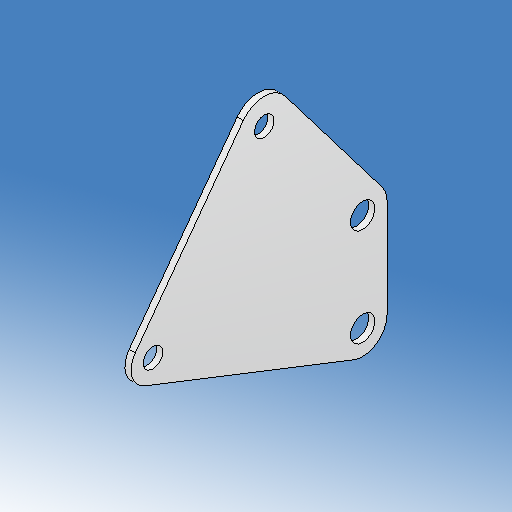
# Autodesk Inventor part: OuterDriveRail
Saved by Autodesk Inventor 2025 (Build 290162000, 162)
## iProperties
Created: 2023-02-06
Part Number: OuterDriveRail
Material: Aluminum 6061
Document SubType Name: Modeling
Designer: kumpu
Density: 2.7 g/cm^3
Appearance: Aluminum - Flat
Mass: 538.586 g
Surface Area: 696.12 cm^2
Volume: 199.476 cm^3
Author: kumpu
Autodesk Inventor part; units mm, degrees
(part 1 of 2)
ref_plane "YZ Plane" through (0, 0, 0) normal (1, 0, 0) x (0, 1, 0)
ref_plane "XZ Plane" through (0, 0, 0) normal (0, 1, 0) x (-1, 0, 0)
ref_plane "XY Plane" through (0, 0, 0) normal (0, 0, 1) x (1, 0, 0)
sketch "Sketch1" plane through (0, 0, 0) normal (1, 0, 0) x (0, 1, 0)
  line L0 (111.125, 190.5) -> (66.5265, 190.5)
  line L1 (19.3212, 158.834) -> (-11.1661, 102.5705)
  arc A0 (-11.1661, 102.5705) -> (-11.1661, 90.4695) centre (0, 96.52) ccw
  line L2 (-11.1661, 90.4695) -> (7.6076, 55.8231)
  arc A1 (-11.1661, 6.0505) -> (-11.1661, -6.0505) centre (0, 0) ccw
  line L3 (-11.1661, -6.0505) -> (7.6076, -40.6969)
  arc A2 (-11.1661, -90.4695) -> (-11.1661, -102.5705) centre (0, -96.52) ccw
  line L4 (-11.1661, -102.5705) -> (19.3212, -158.834)
  line L5 (66.5265, -190.5) -> (111.125, -190.5)
  line L6 (111.125, -190.5) -> (111.125, 190.5)
  arc A3 (19.3212, 158.834) -> (66.5265, 190.5) centre (41.275, 177.125) ccw
  arc A4 (66.5265, -190.5) -> (19.3212, -158.834) centre (41.275, -177.125) ccw
  circle A5 centre (73.5908, -125.0234) radius 6.35 construction
  line L7 (111.125, 0) -> (0, 0) construction
  circle A6 centre (0, 96.52) radius 2.4892 construction
  circle A7 centre (0, 0) radius 2.4892 construction
  circle A8 centre (0, -96.52) radius 2.4892 construction
  line L8 (-11.1661, 6.0505) -> (7.6076, 40.6969)
  arc A9 (7.6076, 40.6969) -> (7.6076, 55.8231) centre (-6.35, 48.26) ccw
  line L9 (-11.1661, -90.4695) -> (7.6076, -55.8231)
  arc A10 (7.6076, -55.8231) -> (7.6076, -40.6969) centre (-6.35, -48.26) ccw
  line L10 (-6.35, -48.26) -> (-6.35, 48.26) construction
  line L11 (-6.35, 0) -> (0, 0) construction
  circle A11 centre (0, 96.52) radius 3.175
  circle A12 centre (0, 0) radius 3.175
  circle A13 centre (0, -96.52) radius 3.175
  circle A14 centre (46.0375, 122.682) radius 3.5687 construction
  circle A15 centre (20.6375, 122.682) radius 3.5687 construction
  circle A16 centre (46.0375, 122.682) radius 3.175
  circle A17 centre (20.6375, 122.682) radius 3.175
  line L12 (0, 96.52) -> (-12.7, 96.52) construction
  circle A18 centre (99.3625, 57.3249) radius 2.0193
  circle A19 centre (48.3094, -33.0391) radius 2.0193
  circle A20 centre (99.3625, 31.9249) radius 2.0193
  circle A21 centre (73.9625, 57.3249) radius 2.0193
  circle A22 centre (73.9625, 31.9249) radius 2.0193
  circle A23 centre (48.3094, -58.4391) radius 2.0193
  circle A24 centre (22.9094, -33.0391) radius 2.0193
  circle A25 centre (22.9094, -58.4391) radius 2.0193
  circle A26 centre (85.725, 107.3629) radius 11
  line L13 (-12.7, 173.6352) -> (-12.7, -210.2893) construction
  circle A27 centre (85.725, 107.3629) radius 17.78 construction
  circle A28 centre (79.375, 147.5038) radius 22.86 construction
  circle A29 centre (41.275, 177.125) radius 25.4 construction
  line L14 (110.475, 71.2949) -> (60.975, 71.2949) construction
  line L15 (60.975, 71.2949) -> (60.975, -72.4091) construction
  line L16 (60.975, -72.4091) -> (110.475, -72.4091) construction
  line L17 (110.475, -72.4091) -> (110.475, 71.2949) construction
  line L18 (59.4219, 71.2949) -> (9.9219, 71.2949) construction
  line L19 (9.9219, 71.2949) -> (9.9219, -72.4091) construction
  line L20 (9.9219, -72.4091) -> (59.4219, -72.4091) construction
  line L21 (59.4219, -72.4091) -> (59.4219, 71.2949) construction
  line L22 (9.525, 127) -> (-15.875, 127) construction
  line L23 (-15.875, 127) -> (-15.875, -177.8) construction
  line L24 (-15.875, -177.8) -> (9.525, -177.8) construction
  line L25 (9.525, -177.8) -> (9.525, 127) construction
  circle A30 centre (34.6719, -108.4771) radius 17.78 construction
  circle A31 centre (41.275, -177.125) radius 31.75 construction
  circle A32 centre (102.0089, 180.2336) radius 2.413
  circle A33 centre (89.3089, 182.1987) radius 2.413
  circle A34 centre (102.0089, -180.2336) radius 2.413
  circle A35 centre (89.3089, -182.1987) radius 2.413
  circle A36 centre (79.375, 147.5038) radius 14.2875
  circle A37 centre (66.675, 254) radius 58.7375 construction
  circle A38 centre (66.675, -254) radius 58.7375 construction
  circle A39 centre (80.899, -155.6385) radius 47.527 construction
  circle A40 centre (92.075, -88.2841) radius 3.175
  circle A41 centre (66.675, -88.2841) radius 3.175
  circle A42 centre (92.075, -88.2841) radius 6.35 construction
  circle A43 centre (66.675, -88.2841) radius 6.35 construction
  circle A44 centre (46.0375, 122.682) radius 6.35 construction
  circle A45 centre (20.6375, 122.682) radius 6.35 construction
  circle A46 centre (17.4625, -132.7341) radius 3.175
  circle A47 centre (17.4625, -132.7341) radius 6.35 construction
  circle A48 centre (103.1875, 79.2324) radius 3.175
  circle A49 centre (103.1875, 79.2324) radius 6.35 construction
  line L26 (92.075, 107.3629) -> (79.375, 107.3629) construction
  line L27 (79.375, 107.3629) -> (79.375, 71.2949) construction
  line L28 (79.375, 71.2949) -> (92.075, 71.2949) construction
  line L29 (92.075, 71.2949) -> (92.075, 107.3629) construction
  line L30 (85.725, 107.3629) -> (85.725, 71.2949) construction
  circle A50 centre (71.4375, 79.2324) radius 3.175
  circle A51 centre (71.4375, 79.2324) radius 6.35 construction
  circle A52 centre (65.2528, -135.2431) radius 22.86 construction
  circle A53 centre (41.275, -177.125) radius 25.4 construction
  circle A54 centre (65.2528, -135.2431) radius 14.2875
  circle A55 centre (41.275, 177.125) radius 22.225 construction
  circle A56 centre (41.275, -177.125) radius 22.225 construction
  circle A57 centre (34.6719, -108.4771) radius 11
  circle A58 centre (79.375, 180.975) radius 3.175
  circle A59 centre (48.1711, 139.457) radius 3.175
  circle A60 centre (20.6375, 144.8678) radius 3.175
  circle A61 centre (79.375, 180.975) radius 6.35 construction
  circle A62 centre (48.1711, 139.457) radius 6.35 construction
  circle A63 centre (20.6375, 144.8678) radius 6.35 construction
  circle A64 centre (41.275, 177.125) radius 38.294 construction
  circle A65 centre (60.325, -104.1591) radius 3.175
  circle A66 centre (60.325, -104.1591) radius 6.35 construction
  point P0 (34.6719, -72.4091)
  dimension "d2" = 15.875
  dimension "d3" = 6.35
  dimension "d4" = 96.52
  dimension "d8" = 6.35
  dimension "d9" = 381
  dimension "d11" = 28.575
  dimension "d12" = 12.7
  dimension "d135" = 4.0386
  dimension "d136" = 4.0386
  dimension "d139" = 25.4
  dimension "d142" = 25.4
  dimension "d147" = 25.4
  dimension "d150" = 25.4
  dimension "d225" = 22
  dimension "d226" = 25.4
  dimension "d227" = 50.038
  dimension "d229" = 123.825
  dimension "d230" = 35.56
  dimension "d231" = 45.72
  dimension "d232" = 50.8
  dimension "d233" = 49.5
  dimension "d234" = 143.704
  dimension "d235" = 13.97
  dimension "d236" = 11.1125
  dimension "d237" = 143.704
  dimension "d238" = 49.5
  dimension "d239" = 11.1125
  dimension "d240" = 13.97
  dimension "d242" = 25.4
  dimension "d243" = 304.8
  dimension "d245" = 9.525
  dimension "d246" = 35.56
  dimension "d248" = 63.5
  dimension "d249" = 28.575
  dimension "d250" = 31.75
  dimension "d251" = 4.826
  dimension "d252" = 4.826
  dimension "d253" = 4.826
  dimension "d254" = 4.826
  dimension "d256" = 9.1161
  dimension "d257" = 12.7
  dimension "d258" = 1.9652
  dimension "d259" = 10.2664
  dimension "d260" = 12.7
  dimension "d261" = 1.9652
  dimension "d262" = 9.1161
  dimension "d263" = 10.2664
  dimension "d264" = 117.475
  dimension "d265" = 117.475
  dimension "d266" = 44.45
  dimension "d267" = 63.5
  dimension "d268" = 63.5
  dimension "d270" = 98.3615
  dimension "d271" = 14.224
  dimension "d272" = 95.054
  dimension "d273" = 6.35
  dimension "d274" = 6.35
  dimension "d275" = 25.4
  dimension "d276" = 19.05
  dimension "d277" = 12.7
  dimension "d278" = 12.7
  dimension "d279" = 12.7
  dimension "d280" = 12.7
  dimension "d283" = 6.35
  constraints: 62 end point, 61 centre point, 30 coincident, 18 point on circle, 17 tangent, 15 equal radius, 10 horizontal, 8 parallel, 6 midpoint, 5 perpendicular, 5 vertical, 2 horizontal alignment, 2 vertical alignment, 1 collinear, 1 equal length, 13 other
  measures "d2" radius of A9
  measures "d3" distance from line of L7.end L10
  measures "d4" distance of L10.start L10.end
  measures "d8" diameter of A11
  measures "d9" distance of L5.end L0.start
  measures "d11" radius of A3
  measures "d12" radius of A0
  measures "d135" diameter of A18
  measures "d136" diameter of A19
  measures "d139" distance of A18.centre A20.centre
  measures "d142" distance of A18.centre A21.centre
  measures "d147" distance of A19.centre A23.centre
  measures "d150" distance of A19.centre A24.centre
  measures "d225" diameter of A26
  measures "d226" distance from line of A26.centre L6
  measures "d227" vertical distance of A21.centre A26.centre
  measures "d229" distance between parallel lines of L13 L6
  measures "d230" diameter of A27
  measures "d231" diameter of A28
  measures "d232" diameter of A29
  measures "d233" distance of L15.end L16.end
  measures "d234" distance of L16.end L14.start
  measures "d235" distance from line of A18.centre L14
  measures "d236" distance from line of L17 A20.centre
  measures "d237" distance of L20.end L18.start
  measures "d238" distance of L18.start L18.end
  measures "d239" distance from line of L21 A23.centre
  measures "d240" distance from line of L20 A25.centre
  measures "d242" distance of L24.end L23.end
  measures "d243" distance of L22.end L23.end
  measures "d245" distance from line of A0.centre L25
  measures "d246" diameter of A30
  measures "d248" diameter of A31
  measures "d249" diameter of A36
  measures "d250" distance from line of A28.centre L6
  measures "d251" diameter of A32
  measures "d252" diameter of A33
  measures "d253" diameter of A34
  measures "d254" diameter of A35
  measures "d256" distance from line of A32.centre L6
  measures "d257" horizontal distance of A33.centre A32.centre
  measures "d258" vertical distance of A33.centre A32.centre
  measures "d259" distance from line of A32.centre L0
  measures "d260" horizontal distance of A35.centre A34.centre
  measures "d261" vertical distance of A35.centre A34.centre
  measures "d262" distance from line of L6 A34.centre
  measures "d263" distance from line of L5 A34.centre
  measures "d264" diameter of A37
  measures "d265" diameter of A38
  measures "d266" distance from line of A37.centre L6
  measures "d267" distance from line of L0 A37.centre
  measures "d268" distance from line of A38.centre L5
  measures "d270" vertical distance of A38.centre A39.centre
  measures "d271" horizontal distance of A38.centre A39.centre
  measures "d272" diameter of A39
  measures "d273" diameter of A41
  measures "d274" diameter of A40
  measures "d275" distance of A41.centre A40.centre
  measures "d276" distance from line of L6 A40.centre
  measures "d277" diameter of A43
  measures "d278" diameter of A42
  measures "d279" diameter of A44
  measures "d280" diameter of A45
  measures "d283" diameter of A46
extrude "Extrusion1" [suppressed]
sketch "Sketch2" plane through (12.7, 0, 0) normal (1, 0, 0) x (0, 0, -1)
  circle A0 centre (-96.52, 0) radius 3.175 construction
  line L0 (190.5, 111.125) -> (-190.5, 111.125) construction
  circle A1 centre (0, 0) radius 3.175 construction
  line L1 (0, 0) -> (0, 111.125) construction
  circle A2 centre (96.52, 0) radius 3.175 construction
  line L2 (96.52, 0) -> (96.52, 111.125) construction
  circle A3 centre (-122.682, 20.6375) radius 3.175 construction
  line L3 (-96.52, 0) -> (-122.682, 20.6375) construction
  circle A4 centre (-122.682, 46.0375) radius 3.175 construction
  line L4 (-122.682, 20.6375) -> (-122.682, 46.0375) construction
  circle A5 centre (-146.05, 85.725) radius 7.9375 construction
  line L5 (-122.682, 46.0375) -> (-146.05, 85.725) construction
  line L6 (-190.5, 111.125) -> (-190.5, 66.5265) construction
  line L7 (-146.05, 85.725) -> (-190.5, 111.125) construction
  line L8 (-146.05, 85.725) -> (-106.0351, 111.125) construction
  circle A6 centre (92.075, 34.925) radius 7.9375 construction
  circle A7 centre (125.0234, 73.5908) radius 6.35 construction
  line L9 (125.0234, 73.5908) -> (92.075, 34.925) construction
  line L10 (125.0234, 73.5908) -> (190.5, 111.125) construction
  line L11 (125.0234, 73.5908) -> (96.52, 111.125) construction
  circle A8 centre (69.85, 100.0125) radius 3.175 construction
  circle A9 centre (69.85, 74.6125) radius 3.175 construction
  line L12 (69.85, 100.0125) -> (69.85, 74.6125) construction
  line L13 (92.075, 34.925) -> (96.52, 0) construction
  line L14 (125.0234, 73.5908) -> (96.52, 0) construction
  line L15 (53.1812, 12.7) -> (53.1812, 57.15) construction
  line L16 (53.1812, 57.15) -> (53.1812, 111.125) construction
  line L17 (69.85, 100.0125) -> (53.1812, 111.125) construction
  line L18 (0, 0) -> (53.1812, 12.7) construction
  line L19 (0, 0) -> (-48.26, 10.3187) construction
  line L20 (-48.26, 10.3187) -> (-96.52, 0) construction
  line L21 (-48.26, 10.3187) -> (0, 111.125) construction
  line L22 (96.52, 0) -> (53.1812, 12.7) construction
  line L23 (-146.05, 85.725) -> (-122.682, 20.6375) construction
  line L24 (190.5, 66.5265) -> (190.5, 111.125) construction
  circle A10 centre (-190.5, 111.125) radius 3.9688 construction
  circle A11 centre (-96.52, 0) radius 3.9688 construction
  circle A12 centre (0, 0) radius 3.9688 construction
  circle A13 centre (96.52, 0) radius 3.9688 construction
  circle A14 centre (190.5, 111.125) radius 3.9688 construction
  circle A15 centre (0, 111.125) radius 3.9688 construction
  circle A16 centre (-146.05, 85.725) radius 3.9688 construction
  circle A17 centre (125.0234, 73.5908) radius 3.9688 construction
  circle A18 centre (92.075, 34.925) radius 3.9688 construction
  circle A19 centre (-48.26, 10.3187) radius 3.9688 construction
  circle A20 centre (-106.0351, 111.125) radius 3.9688 construction
  line L25 (-136.5891, 96.4312) -> (-119.693, 107.1562)
  line L26 (-119.693, 107.1562) -> (-167.6665, 107.1562)
  line L27 (-65.4177, 107.1562) -> (-6.3001, 107.1562)
  line L28 (-6.3001, 107.1562) -> (-48.5749, 18.852)
  line L29 (3.9688, 107.1562) -> (49.2625, 107.1562)
  line L30 (49.2625, 107.1562) -> (49.2625, 59.3278)
  line L31 (104.5173, 107.1562) -> (120.8881, 85.5986)
  line L32 (168.255, 107.1562) -> (104.5173, 107.1562)
  circle A21 centre (96.52, 111.125) radius 3.9688 construction
  circle A22 centre (69.85, 100.0125) radius 3.9688 construction
  circle A23 centre (69.85, 74.6125) radius 3.9688 construction
  line L33 (-132.3353, 89.7298) -> (-108.668, 104.7529)
  line L34 (-119.4185, 54.986) -> (-101.1904, 73.4311)
  circle A24 centre (-122.682, 46.0375) radius 3.9688 construction
  circle A25 centre (-122.682, 20.6375) radius 3.9688 construction
  circle A26 centre (-122.682, 46.0375) radius 9.525 construction
  line L35 (-3.9688, 93.644) -> (-42.0864, 14.0232)
  line L36 (-3.9688, 10.3796) -> (-3.9688, 93.644)
  line L37 (3.9688, 107.1562) -> (3.9688, 11.314)
  circle A27 centre (0, 0) radius 3.175 projected
  line L38 (73.7765, 65.9345) -> (112.3781, 74.7683)
  line L39 (77.1781, 80.6973) -> (96.4328, 104.6775)
  line L40 (96.4328, 104.6775) -> (114.5667, 80.7982)
  line L41 (63.9805, 55.55) -> (114.1488, 67.0308)
  line L42 (82.1272, 45.1805) -> (63.9805, 55.55)
  line L43 (89.8709, 20.8085) -> (91.2725, 9.7955)
  line L44 (-122.682, 46.0375) -> (-76.4287, 92.8415) construction
  line L45 (-190.5, 111.125) -> (-190.5, -12.7)
  line L46 (-190.5, -12.7) -> (190.5, -12.7)
  line L47 (190.5, -12.7) -> (190.5, 111.125)
  arc A28 (-6.0505, -11.1661) -> (6.0505, -11.1661) centre (0, 0) ccw construction
  arc A29 (-136.5891, 96.4312) -> (-156.4804, 95.4891) centre (-146.05, 85.725) ccw
  arc A30 (-131.772, 86.2463) -> (-132.3353, 89.7298) centre (-146.05, 85.725) ccw
  arc A31 (-190.5, 111.125) -> (-184.6538, 104.795) centre (-184.15, 111.125) ccw
  arc A32 (-160.0618, 82.9318) -> (-184.6538, 104.795) centre (-186.8185, 77.5979) ccw
  arc A33 (-160.0618, 82.9318) -> (-153.0864, 73.2903) centre (-146.05, 85.725) ccw
  arc A34 (-131.8934, 23.0615) -> (-153.0864, 73.2903) centre (-175.0785, 34.4258) ccw
  arc A35 (-119.4185, 54.986) -> (-126.5651, 54.735) centre (-122.682, 46.0375) ccw
  arc A36 (-131.8934, 23.0615) -> (-118.8104, 11.9348) centre (-122.682, 20.6375) ccw
  arc A37 (-156.4804, 95.4891) -> (-167.6665, 107.1562) centre (-186.8185, 77.5979) ccw
  arc A38 (-126.5651, 54.735) -> (-139.486, 73.1451) centre (-175.0785, 34.4258) ccw
  arc A39 (-139.486, 73.1451) -> (-133.8392, 78.5818) centre (-146.192, 85.761) ccw
  line L48 (-96.52, 0) -> (0, 0) construction
  line L49 (-48.26, 0) -> (-48.26, 6.35) construction
  arc A40 (-107.3496, 2.4916) -> (-118.8104, 11.9348) centre (-115.4372, 4.3524) ccw
  arc A41 (-107.3496, 2.4916) -> (-89.4091, -8.5395) centre (-96.52, 0) ccw
  arc A42 (-7.1109, -8.5395) -> (-89.4091, -8.5395) centre (-48.26, -57.9553) ccw
  arc A43 (-7.1109, -8.5395) -> (7.1109, -8.5395) centre (0, 0) ccw
  arc A44 (89.4091, -8.5395) -> (7.1109, -8.5395) centre (48.26, -57.9553) ccw
  arc A45 (89.4091, -8.5395) -> (107.4129, 2.1985) centre (96.52, 0) ccw
  arc A46 (132.1844, 63.1022) -> (107.4129, 2.1985) centre (165.7303, 13.9684) ccw
  arc A47 (185.7041, 104.9681) -> (190.5, 111.125) centre (184.15, 111.125) ccw
  arc A48 (185.7041, 104.9681) -> (136.0465, 67.2834) centre (205.2058, 27.7108) ccw
  arc A49 (132.1844, 63.1022) -> (136.0465, 67.2834) centre (125.0234, 73.5908) ccw
  arc A50 (-86.0187, 3.6345) -> (-88.1432, 7.3019) centre (-96.52, 0) ccw
  arc A51 (-3.9688, 10.3796) -> (-10.5013, 3.6345) centre (0, 0) ccw
  arc A52 (-10.5013, 3.6345) -> (-42.0864, 14.0232) centre (-48.26, -57.9553) ccw
  arc A53 (-53.8119, 14.0739) -> (-86.0187, 3.6345) centre (-48.26, -57.9553) ccw
  arc A54 (10.5013, 3.6345) -> (9.5832, 5.6259) centre (0, 0) ccw
  arc A55 (39.4872, 13.7529) -> (10.5013, 3.6345) centre (48.26, -57.9553) ccw
  arc A56 (86.0187, 3.6345) -> (47.4247, 14.2827) centre (48.26, -57.9553) ccw
  arc A57 (91.2725, 9.7955) -> (86.0187, 3.6345) centre (96.52, 0) ccw
  arc A58 (135.4904, 80.7834) -> (120.8881, 85.5986) centre (125.0234, 73.5908) ccw
  arc A59 (168.255, 107.1562) -> (135.4904, 80.7834) centre (205.2058, 27.7108) ccw
  arc A60 (73.7765, 65.9345) -> (77.1781, 80.6973) centre (69.85, 74.6125) ccw
  arc A61 (114.5667, 80.7982) -> (112.3781, 74.7683) centre (125.0234, 73.5908) ccw
  arc A62 (101.052, 46.0401) -> (82.1272, 45.1805) centre (92.075, 34.925) ccw
  arc A63 (79.7883, 42.2168) -> (80.2054, 26.9722) centre (92.075, 34.925) ccw
  arc A64 (80.2054, 26.9722) -> (89.8709, 20.8085) centre (92.075, 34.925) ccw
  arc A65 (114.1488, 67.0308) -> (115.2054, 65.5349) centre (125.0234, 73.5908) ccw
  arc A66 (115.2054, 65.5349) -> (101.052, 46.0401) centre (165.7303, 13.9684) ccw
  circle A67 centre (-57.3249, 99.3625) radius 2.0193 construction
  circle A68 centre (-57.3249, 73.9625) radius 2.0193 construction
  circle A69 centre (-31.9249, 99.3625) radius 2.0193 construction
  circle A70 centre (-31.9249, 73.9625) radius 2.0193 construction
  circle A71 centre (58.4391, 22.9094) radius 2.0193 construction
  circle A72 centre (33.0391, 22.9094) radius 2.0193 construction
  circle A73 centre (33.0391, 48.3094) radius 2.0193 construction
  circle A74 centre (58.4391, 48.3094) radius 2.0193 construction
  line L50 (-106.0351, 111.125) -> (-81.6196, 80.1887) construction
  line L51 (-96.012, 99.3625) -> (-96.012, 73.9625) construction
  line L52 (-57.3249, 73.025) -> (-31.9249, 73.025) construction
  line L53 (-70.612, 73.9625) -> (-70.612, 99.3625) construction
  line L54 (-31.9249, 98.425) -> (-57.3249, 98.425) construction
  line L55 (-146.192, 85.761) -> (-59.8898, 63.8569) construction
  line L56 (-96.0036, 74.2316) -> (-96.52, 0) construction
  line L57 (-96.52, 0) -> (-65.9914, 86.0487) construction
  circle A75 centre (-57.3249, 99.3625) radius 5.1943
  circle A76 centre (-70.612, 98.425) radius 5.1943
  circle A77 centre (-96.012, 73.025) radius 5.1943
  circle A78 centre (-70.612, 73.025) radius 5.1943
  circle A79 centre (33.0391, 48.3094) radius 5.1943
  circle A80 centre (43.18, 47.625) radius 5.1943
  circle A81 centre (17.78, 22.225) radius 5.1943
  circle A82 centre (43.18, 22.225) radius 5.1943
  line L58 (-70.612, 73.025) -> (-48.26, 10.3187) construction
  line L59 (-99.4531, 94.4823) -> (-108.668, 104.7529)
  line L60 (-133.8392, 78.5818) -> (-100.2798, 70.0642)
  line L61 (-131.772, 86.2463) -> (-98.2146, 77.7292)
  line L62 (-77.1372, 79.5502) -> (-70.612, 73.025) construction
  line L63 (-92.6609, 76.9937) -> (-73.9631, 76.9937)
  line L64 (-92.6609, 69.0562) -> (-73.9631, 69.0562)
  line L65 (-74.5808, 95.0739) -> (-74.5808, 76.3761)
  line L66 (-66.6433, 95.0739) -> (-66.6433, 76.3761)
  line L67 (-99.9808, 95.0739) -> (-99.9808, 76.3761)
  line L68 (-92.0433, 95.0739) -> (-92.0433, 76.3761)
  line L69 (-92.6609, 94.4562) -> (-73.9631, 94.4562)
  line L70 (-92.6609, 102.3937) -> (-73.9631, 102.3937)
  line L71 (-96.4488, 93.2491) -> (-75.7879, 72.5882)
  line L72 (-90.8361, 98.8618) -> (-70.1752, 78.2009)
  line L73 (-113.7728, 49.4066) -> (-95.5446, 67.8518)
  line L74 (-73.2252, 68.5359) -> (-53.8119, 14.0739)
  line L75 (-65.7485, 71.201) -> (-47.7228, 20.6319)
  line L76 (-89.3091, 8.4552) -> (-67.9922, 68.5398)
  line L77 (-96.7898, 11.1092) -> (-75.4728, 71.1938)
  line L78 (-100.2104, 20.4213) -> (-100.2104, 69.9665)
  line L79 (-92.4791, 10.3518) -> (-92.0667, 69.6464)
  line L80 (-113.5349, 43.3812) -> (-100.2104, 20.4213)
  arc A83 (-113.5349, 43.3812) -> (-113.7728, 49.4066) centre (-122.682, 46.0375) ccw
  circle A84 centre (-96.52, 0) radius 11.1125 construction
  arc A85 (-88.1432, 7.3019) -> (-89.3091, 8.4552) centre (-96.52, 0) ccw
  line L81 (-65.4177, 107.1562) -> (-65.4177, 98.425)
  line L82 (17.78, 22.225) -> (43.18, 22.225) construction
  line L83 (43.18, 22.225) -> (43.18, 47.625) construction
  line L84 (43.18, 47.625) -> (33.0391, 47.625) construction
  line L85 (17.78, 48.3094) -> (17.78, 22.225) construction
  line L86 (25.0718, 40.3375) -> (43.1946, 22.225) construction
  line L87 (17.78, 22.225) -> (0, 0) construction
  line L88 (69.85, 74.6125) -> (43.18, 47.625) construction
  line L89 (92.075, 34.925) -> (43.18, 47.625) construction
  line L90 (92.075, 34.925) -> (43.1946, 22.225) construction
  line L91 (21.1311, 51.5938) -> (39.8289, 51.5938)
  line L92 (21.1311, 43.6563) -> (39.8289, 43.6563)
  line L93 (13.8112, 44.2739) -> (13.8112, 25.4502)
  line L94 (12.5875, 22.0875) -> (-3.0991, 2.4793)
  line L95 (18.7857, 17.129) -> (3.0991, -2.4793)
  line L96 (21.1311, 18.2563) -> (39.8289, 18.2563)
  line L97 (21.1311, 26.1938) -> (39.8289, 26.1938)
  line L98 (39.2112, 25.5761) -> (39.2112, 44.2739)
  line L99 (47.1487, 25.5761) -> (47.1487, 44.2739)
  line L100 (43.6313, 27.3997) -> (22.9558, 48.0632)
  line L101 (38.0029, 21.8027) -> (17.3447, 42.449)
  line L102 (67.0195, 77.3945) -> (42.8556, 52.8092)
  line L103 (48.3446, 47.0702) -> (72.6805, 71.8305)
  line L104 (45.4257, 42.9413) -> (77.7928, 34.5342)
  line L105 (47.4212, 50.6238) -> (79.7883, 42.2168) construction
  line L106 (46.5311, 18.2563) -> (80.1865, 27.0005)
  line L107 (45.4305, 26.9064) -> (77.7928, 35.3147)
  line L108 (21.7487, 44.2739) -> (21.7487, 25.5761)
  line L109 (14.4289, 51.5938) -> (3.9688, 51.5938)
  line L110 (14.4289, 43.6563) -> (3.9688, 43.6563)
  line L111 (33.0391, 47.625) -> (0, 47.625) construction
  line L112 (39.4872, 18.5721) -> (39.4872, 8.9337)
  line L113 (47.4247, 19.2311) -> (47.4247, 9.3342)
  point P0 (-104.0605, 99.6176)
  point P1 (-83.312, 76.9937)
  point P2 (-74.5808, 85.725)
  point P3 (-104.6587, 58.6292)
  point P4 (-110.3045, 64.2086)
  point P5 (-109.347, 59.5312)
  point P6 (-92.2729, 39.9991)
  point P7 (-103.6679, 70.9241)
  point P8 (-70.6032, 61.1802)
  point P9 (-92.0708, 69.0562)
  point P10 (-92.3876, 23.5174)
  point P11 (-76.2312, 69.0562)
  point P12 (-100.2104, 63.1305)
  point P13 (-99.9808, 78.1775)
  point P14 (-99.9808, 95.0704)
  point P15 (-86.4306, 94.4562)
  point P16 (-74.5808, 82.6064)
  point P17 (-74.5808, 94.4562)
  point P18 (-80.1934, 76.9937)
  point P19 (-92.0433, 88.8436)
  point P20 (-92.0433, 76.9937)
  point P21 (30.48, 51.5938)
  point P22 (33.2935, 37.7315)
  point P23 (39.2112, 34.925)
  point P24 (9.1988, 43.6563)
  point P25 (0, 47.625)
  point P26 (47.1487, 27.3529)
  point P27 (76.2905, 34.9244)
  point P28 (47.1487, 42.4937)
  point P29 (39.4872, 18.2563)
  point P30 (27.3653, 43.6563)
  point P31 (39.2112, 31.8171)
  point P32 (39.2112, 43.6563)
  point P33 (21.7487, 38.0475)
  point P34 (21.7487, 26.1938)
  point P35 (33.6093, 26.1938)
  point P36 (13.8112, 43.6563)
  point P37 (13.8112, 25.5761)
  point P38 (47.4247, 18.4884)
  dimension "d17" = 19.05
  dimension "d65" = 12.7
  dimension "d13" = 44.45
  dimension "d14" = 7.9375
  dimension "d29" = 14.2875
  dimension "d30" = 9.525
  dimension "d31" = 6.35
  dimension "d32" = 7.9375
  dimension "d33" = 7.9375
  dimension "d34" = 6.35
  dimension "d35" = 11.1125
  dimension "d36" = 12.7
  dimension "d37" = 7.9375
  dimension "d38" = 7.9375
  dimension "d39" = 7.9375
  dimension "d40" = 12.7
  dimension "d157" = 3.175
  dimension "d160" = 25.4
  dimension "d163" = 25.4
  dimension "d166" = 3.175
  dimension "d169" = 25.4
  dimension "d172" = 25.4
  dimension "d177" = 7.9375
  dimension "d180" = 7.9375
  dimension "d181" = 3.9688
  dimension "d182" = 7.9375
  dimension "d183" = 3.9688
  dimension "d185" = 7.9375
  dimension "d186" = 3.9688
  dimension "d187" = 7.9375
  dimension "d188" = 3.9688
  dimension "d189" = 7.9375
  dimension "d190" = 3.9688
  dimension "d191" = 7.9375
  dimension "d192" = 3.9688
  dimension "d194" = 7.9375
  dimension "d195" = 7.9375
  dimension "d196" = 3.9688
  dimension "d197" = 3.9688
  dimension "d198" = 7.9375
  dimension "d199" = 3.9688
  dimension "d202" = 7.9375
  dimension "d203" = 0.156
  dimension "d204" = 7.9375
  dimension "d205" = 3.9688
  dimension "d206" = 7.9375
  dimension "d207" = 3.9688
  dimension "d208" = 7.9375
  dimension "d209" = 3.9688
  dimension "d210" = 7.9375
  dimension "d211" = 7.9375
  dimension "d212" = 3.9688
  dimension "d213" = 3.9688
  dimension "d214" = 3.9688
  dimension "d215" = 8.649
  dimension "d216" = 3.9688
  dimension "d217" = 7.9375
  dimension "d218" = 3.9688
  dimension "d220" = 7.9375
  dimension "d221" = 7.9375
  dimension "d222" = 3.9688
  dimension "d223" = 7.9375
  constraints: 222 end point, 104 point on circle, 59 centre point, 42 tangent, 33 concentric, 33 parallel, 28 coincident, 22 equal radius, 18 vertical, 14 midpoint, 14 point on line, 13 horizontal, 13 perpendicular, 3 collinear, 2 line through centre, 1 equal length, 82 other
  measures "d13" distance of L15.start L15.end
  measures "d14" diameter of A10
  measures "d29" radius of A29
  measures "d30" radius of A35
  measures "d31" radius of A31
  measures "d32" radial gap between concentric circles of A32 A37
  measures "d33" radial gap between concentric circles of A34 A38
  measures "d34" distance of L49.start L49.end
  measures "d35" radius of A41
  measures "d36" radius of A49
  measures "d37" radial gap between concentric circles of A42 A53
  measures "d38" radial gap between concentric circles of A44 A55
  measures "d39" radial gap between concentric circles of A48 A59
  measures "d40" radial gap between concentric circles of A46 A66
  measures "d177" distance between parallel lines of L61 L60
  measures "d180" distance from line of L64 point (-83.312, 76.994)
  measures "d181" distance between parallel lines of L63 L52
  measures "d182" distance between parallel lines of L66 L65
  measures "d183" distance from line of point (-74.581, 85.725) L53
  measures "d185" distance between parallel lines of L68 L67
  measures "d186" distance between parallel lines of L67 L51
  measures "d187" distance between parallel lines of L69 L70
  measures "d188" distance between parallel lines of L54 L70
  measures "d189" distance between parallel lines of L72 L71
  measures "d190" distance between parallel lines of L62 L71
  measures "d191" distance of point (-104.659, 58.629) point (-110.304, 64.209)
  measures "d192" distance from line of L73 point (-109.347, 59.531)
  measures "d194" distance from line of point (-92.273, 39.999) L78
  measures "d195" distance between parallel lines of L76 L77
  measures "d196" distance between parallel lines of L79 L56
  measures "d197" distance between parallel lines of L76 L57
  measures "d198" distance between parallel lines of L75 L74
  measures "d199" distance between parallel lines of L58 L74
  measures "d202" distance between parallel lines of L103 L102
  measures "d203" angle of L102 L88
  measures "d204" distance from line of L92 point (30.48, 51.594)
  measures "d205" distance between parallel lines of L91 L84
  measures "d206" distance between parallel lines of L100 L101
  measures "d207" distance from line of point (33.294, 37.731) L86
  measures "d208" distance between parallel lines of L108 L93
  measures "d209" distance between parallel lines of L108 L85
  measures "d210" distance from line of L99 point (39.211, 34.925)
  measures "d211" distance between parallel lines of L96 L97
  measures "d212" distance between parallel lines of L82 L96
  measures "d213" distance between parallel lines of L99 L83
  measures "d214" distance between parallel lines of L107 L90
  measures "d215" distance between parallel lines of L107 L106
  measures "d216" distance between parallel lines of L89 L104
  measures "d217" distance between parallel lines of L105 L104
  measures "d218" distance between parallel lines of L87 L94
  measures "d220" distance between parallel lines of L95 L94
  measures "d221" distance from line of L109 point (9.199, 43.656)
  measures "d222" distance between parallel lines of L110 L111
  measures "d223" horizontal distance of A56.end A55.start
extrude "Extrusion2" [suppressed]
delete_face "Delete Face1" [suppressed]
fillet "Fillet1" [suppressed]
fillet "Fillet2" [suppressed]
fillet "Fillet3" [suppressed]
sketch "Sketch4" plane through (0, 111.125, 190.5) normal (0, 1, 0) x (1, 0, 0)
  line L0 (12.7, 281.8419) -> (12.7, 291.8504) projected
  line L1 (12.7, 346.4492) -> (12.7, 349.6242) projected
  line L2 (12.7, 26.0204) -> (12.7, 27.6079) projected
  line L3 (12.7, 381) -> (12.7, 0) projected
  line L4 (12.7, 18.9559) -> (0, 18.9559)
  line L5 (12.7, 87.1601) -> (0, 87.1601)
  line L6 (0, 381) -> (0, 0) projected
  line L7 (12.7, 190.5) -> (0, 190.5)
  line L8 (12.7, 274.2219) -> (0, 274.2219)
  line L9 (12.7, 357.5617) -> (0, 357.5617)
  circle A0 centre (6.35, 18.9559) radius 3.175
  circle A1 centre (6.35, 87.1601) radius 3.175
  circle A2 centre (6.35, 190.5) radius 3.175
  circle A3 centre (6.35, 274.2219) radius 3.175
  circle A4 centre (6.35, 357.5617) radius 3.175
  point P0 (12.7, 194.4688)
  point P1 (12.7, 186.5313)
  point P2 (12.7, 80.518)
  point P3 (12.7, 94.0577)
  point P4 (12.7, 348.1717)
  point P5 (12.7, 26.5759)
  point P6 (12.7, 348.0367)
  dimension "d42" = 9.525
  dimension "d43" = 7.62
  dimension "d44" = 6.6421
  dimension "d45" = 7.62
  dimension "d46" = 6.35
  dimension "d47" = 6.35
  dimension "d48" = 6.35
  dimension "d49" = 6.35
  dimension "d50" = 6.35
  constraints: 10 end point, 6 midpoint, 5 centre point, 3 horizontal, 2 point on line, 1 parallel, 1 perpendicular, 6 other
  measures "d42" distance from line of point (12.7, 348.037) L9
  measures "d43" distance from line of L0.start L8
  measures "d44" distance from line of L5 point (12.7, 80.518)
  measures "d45" distance from line of point (12.7, 26.576) L4
  measures "d46" diameter of A0
  measures "d47" diameter of A1
  measures "d48" diameter of A2
  measures "d49" diameter of A3
  measures "d50" diameter of A4
extrude "Extrusion4" [suppressed]
thread "Thread1" size "1/4-20 UNC" class "2B" standard "ANSI Unified Screw Threads" full length
thread "Thread2" size "1/4-20 UNC" class "2B" standard "ANSI Unified Screw Threads" full length
thread "Thread3" size "1/4-20 UNC" class "2B" standard "ANSI Unified Screw Threads" full length
thread "Thread4" size "1/4-20 UNC" class "2B" standard "ANSI Unified Screw Threads" full length
thread "Thread5" size "1/4-20 UNC" class "2B" standard "ANSI Unified Screw Threads" full length
sketch "Sketch5" plane through (12.7, 111.125, 190.5) normal (1, 0, 0) x (0, 0, -1)
  arc A0 (0, 0) -> (5.8462, -6.33) centre (6.35, 0) ccw projected
  arc A1 (30.4382, -28.1932) -> (37.4136, -37.8347) centre (44.45, -25.4) ccw projected
  arc A2 (58.6066, -88.0635) -> (37.4136, -37.8347) centre (15.4215, -76.6992) ccw projected
  spline S0 degree 4 poles (0, 0) (0, -17.1941) (-2.2287, -33.2158) (22.5292, -29.4121) (37.4136, -37.8347) knots 0 0 0 0 0 1 1 1 1 1
  line L0 (0, 8.2432) -> (0, -8.2432) construction
  arc A3 (-0.1228, -6.59) -> (-0.1228, 6.59) centre (-176.868, 0) ccw construction
  line L1 (31.1102, -34.2678) -> (43.7171, -41.4016) construction
  arc A4 (42.0116, -41.1741) -> (32.1834, -35.6126) centre (25.0253, -59.7274) ccw construction
  arc A5 (30.4382, -28.1932) -> (5.8462, -6.33) centre (3.6815, -33.5271) ccw projected
  point P0 (190.5, -111.125)
  point P1 (5.8462, -25.4)
  constraints: 4 end point, 4 midpoint, 2 centre point, 2 point on circle, 2 vertical, 1 tangent, 6 other
extrude "Extrusion5" [suppressed]
sketch "Sketch6" plane through (12.7, -57.9553, 48.26) normal (1, 0, 0) x (0, 0, -1)
  arc A0 (-123.1359, 156.0289) -> (-125.9731, 144.465) centre (-97.79, 143.6803) ccw
  line L0 (-122.8964, 163.3325) -> (-122.523, 159.4124)
  line L1 (-142.24, 169.0803) -> (-129.2178, 169.0803)
  spline S0 degree 2 poles (-221.2962, 144.7093) (-189.8396, 169.0803) (-142.24, 169.0803) knots 1 1 1 2 2 2
  arc A1 (-221.2962, 144.7093) -> (-187.7795, 106.6698) centre (-205.74, 124.6303) ccw
  circle A2 centre (-133.9387, 147.2642) radius 6.35
  line L2 (-141.6133, 153.8382) -> (-140.1827, 146.1086)
  line L3 (-135.7752, 141.1856) -> (-124.621, 137.8157)
  line L4 (238.76, 169.0803) -> (-142.24, 169.0803)
  circle A3 centre (144.78, 57.9553) radius 3.175
  circle A4 centre (-48.26, 57.9553) radius 3.175
  circle A5 centre (48.26, 57.9553) radius 3.175
  circle A6 centre (-74.422, 103.9928) radius 3.175
  circle A7 centre (-74.422, 78.5928) radius 3.175
  spline S1 degree 3 poles (-159.7966, 136.4204) (-160.5161, 136.0307) (-162.9434, 134.6743) (-166.1744, 132.6857) (-170.3078, 129.9138) (-173.1321, 127.8669) (-175.1101, 126.3517) (-175.4939, 126.0547) knots 0 0 0 0 0.132459 0.448869 0.607074 0.923484 1 1 1 1
  spline S2 degree 3 poles (-180.582, 128.1282) (-180.5251, 127.7187) (-180.3887, 127.3243) (-179.9724, 126.6098) (-179.6965, 126.2967) (-179.0402, 125.7938) (-178.666, 125.6088) (-177.8679, 125.3927) (-177.4515, 125.3637) (-176.7607, 125.4505) (-176.4861, 125.5231) (-175.9633, 125.7391) (-175.7175, 125.8816) (-175.4939, 126.0547) knots 0 0 0 0 0.12403 0.12403 0.248059 0.248059 0.372089 0.372089 0.496118 0.496118 0.580963 0.580963 0.665808 0.665808 0.665808 0.665808
  arc A8 (-180.582, 128.1282) -> (-185.3963, 139.8386) centre (-205.74, 124.6303) ccw
  arc A9 (-182.4834, 144.893) -> (-185.3963, 139.8386) centre (-182.8533, 141.7397) ccw
  line L5 (-182.4834, 144.893) -> (-160.9387, 142.3656)
  spline S3 degree 3 poles (-159.7966, 136.4204) (-159.4331, 136.6173) (-159.1114, 136.8833) (-158.5883, 137.5236) (-158.3918, 137.8918) (-158.1509, 138.6828) (-158.1089, 139.0981) (-158.1864, 139.9213) (-158.3051, 140.3214) (-158.6893, 141.0536) (-158.9511, 141.3786) (-159.5039, 141.8425) (-159.7675, 142.0051) (-160.3334, 142.2494) (-160.6326, 142.3297) (-160.9387, 142.3656) knots 0 0 0 0 0.12403 0.12403 0.248059 0.248059 0.372089 0.372089 0.496118 0.496118 0.620148 0.620148 0.712599 0.712599 0.80505 0.80505 0.80505 0.80505
  line L6 (-150.5941, 147.5473) -> (-181.7868, 151.2066)
  spline S4 degree 3 poles (-182.3079, 157.4074) (-182.7047, 157.2914) (-183.0751, 157.099) (-183.7212, 156.583) (-183.9908, 156.2643) (-184.3926, 155.5417) (-184.521, 155.1446) (-184.6185, 154.3235) (-184.5865, 153.9073) (-184.3649, 153.1107) (-184.1773, 152.7379) (-183.6699, 152.085) (-183.3548, 151.8113) (-182.8106, 151.4993) (-182.6148, 151.4119) (-182.2086, 151.2779) (-181.9992, 151.2315) (-181.7868, 151.2066) knots 0 0 0 0 0.12403 0.12403 0.248059 0.248059 0.372089 0.372089 0.496118 0.496118 0.620148 0.620148 0.744178 0.744178 0.808342 0.808342 0.872507 0.872507 0.872507 0.872507
  spline S5 degree 3 poles (-182.3079, 157.4074) (-181.8014, 157.5555) (-180.2373, 158.0014) (-176.5127, 158.9811) (-172.1175, 159.9481) (-165.3484, 161.1597) (-158.303, 162.0566) (-152.1732, 162.4641) (-149.655, 162.5727) knots 0 0 0 0 0.050647 0.155729 0.365894 0.470976 0.786223 1 1 1 1
  spline S6 degree 3 poles (-146.3536, 159.1439) (-146.3201, 159.5559) (-146.3675, 159.9706) (-146.6185, 160.7584) (-146.8198, 161.1241) (-147.3511, 161.7576) (-147.6761, 162.0195) (-148.2892, 162.3414) (-148.5523, 162.438) (-149.097, 162.5599) (-149.3762, 162.5847) (-149.655, 162.5727) knots 0 0 0 0 0.12403 0.12403 0.248059 0.248059 0.372089 0.372089 0.45581 0.45581 0.539531 0.539531 0.539531 0.539531
  line L7 (-146.3536, 159.1439) -> (-147.0595, 150.4439)
  arc A10 (-150.5941, 147.5473) -> (-147.0595, 150.4439) centre (-150.2241, 150.7007) ccw
  arc A11 (-122.8964, 163.3325) -> (-129.2178, 169.0803) centre (-129.2178, 162.7303) ccw
  spline S7 degree 3 poles (-125.9731, 144.465) (-125.9961, 143.6384) (-126.1803, 142.8243) (-126.8505, 141.3124) (-127.33, 140.6292) (-128.4917, 139.516) (-129.1514, 139.0838) (-130.5947, 138.4809) (-131.3658, 138.3154) (-132.1476, 138.2941) knots 0 0 0 0 0.248059 0.248059 0.496118 0.496118 0.730735 0.730735 0.965351 0.965351 0.965351 0.965351
  arc A12 (-123.1359, 156.0289) -> (-122.523, 159.4124) centre (-128.8444, 158.8102) ccw
  spline S8 degree 3 poles (-132.1476, 138.2941) (-151.3774, 137.7699) (-171.7443, 122.7049) (-187.7795, 106.6698) knots 0.172109 0.172109 0.172109 0.172109 1 1 1 1
  circle A13 centre (-205.74, 124.6303) radius 15.24
  circle A14 centre (-133.9387, 147.2642) radius 1.27
  circle A15 centre (-131.9736, 159.9642) radius 1.27
  circle A16 centre (81.2991, 80.8647) radius 2.0193
  line L8 (-142.24, 169.0803) -> (-142.24, 124.4818)
  arc A17 (-110.574, 77.2765) -> (-142.24, 124.4818) centre (-128.865, 99.2303) ccw
  line L9 (-110.574, 77.2765) -> (-54.3105, 46.7892)
  arc A18 (-54.3105, 46.7892) -> (-42.2095, 46.7892) centre (-48.26, 57.9553) ccw
  line L10 (-42.2095, 46.7892) -> (-7.5631, 65.5629)
  arc A19 (7.5631, 65.5629) -> (-7.5631, 65.5629) centre (0, 51.6053) ccw
  line L11 (7.5631, 65.5629) -> (42.2095, 46.7892)
  arc A20 (42.2095, 46.7892) -> (54.3105, 46.7892) centre (48.26, 57.9553) ccw
  line L12 (54.3105, 46.7892) -> (88.9569, 65.5629)
  arc A21 (104.0831, 65.5629) -> (88.9569, 65.5629) centre (96.52, 51.6053) ccw
  line L13 (104.0831, 65.5629) -> (138.7295, 46.7892)
  arc A22 (138.7295, 46.7892) -> (150.8305, 46.7892) centre (144.78, 57.9553) ccw
  line L14 (150.8305, 46.7892) -> (207.094, 77.2765)
  arc A23 (238.76, 124.4818) -> (207.094, 77.2765) centre (225.385, 99.2303) ccw
  line L15 (238.76, 124.4818) -> (238.76, 169.0803)
  circle A24 centre (-99.2438, 137.3303) radius 14.2875
  point P0 (-132.6841, 141.0394)
  point P1 (-140.0973, 148.8119)
  dimension "d65" = 12.7
  constraints: 4 end point, 2 point on circle, 2 tangent, 1 centre point, 4 other
  measures "d65" diameter of A2
extrude "Extrusion6" [suppressed]
sketch "Sketch7" plane through (12.7, -57.9553, 48.26) normal (1, 0, 0) x (0, 0, -1)
  line L0 (238.76, 169.0803) -> (-142.24, 169.0803) projected
  circle A0 centre (144.78, 57.9553) radius 3.175 projected
  circle A1 centre (-48.26, 57.9553) radius 3.175 projected
  circle A2 centre (48.26, 57.9553) radius 3.175 projected
  circle A3 centre (-74.422, 103.9928) radius 3.175 projected
  circle A4 centre (-74.422, 78.5928) radius 3.175 projected
  arc A5 (-140.0973, 148.8119) -> (-132.6841, 141.0394) centre (-133.9387, 147.2642) ccw projected
  line L1 (-135.7752, 141.1856) -> (-124.621, 137.8157)
  line L2 (-141.4444, 152.9909) -> (-140.1846, 146.1192)
  circle A6 centre (81.2991, 80.8647) radius 2.0193 projected
  line L3 (-142.24, 169.0803) -> (-142.24, 124.4818) projected
  arc A7 (-110.574, 77.2765) -> (-142.24, 124.4818) centre (-128.865, 99.2303) ccw projected
  line L4 (-110.574, 77.2765) -> (-54.3105, 46.7892) projected
  arc A8 (-54.3105, 46.7892) -> (-42.2095, 46.7892) centre (-48.26, 57.9553) ccw projected
  line L5 (-42.2095, 46.7892) -> (-7.5631, 65.5629) projected
  arc A9 (7.5631, 65.5629) -> (-7.5631, 65.5629) centre (0, 51.6053) ccw projected
  line L6 (7.5631, 65.5629) -> (42.2095, 46.7892) projected
  arc A10 (42.2095, 46.7892) -> (54.3105, 46.7892) centre (48.26, 57.9553) ccw projected
  line L7 (54.3105, 46.7892) -> (88.9569, 65.5629) projected
  arc A11 (104.0831, 65.5629) -> (88.9569, 65.5629) centre (96.52, 51.6053) ccw projected
  line L8 (104.0831, 65.5629) -> (138.7295, 46.7892) projected
  arc A12 (138.7295, 46.7892) -> (150.8305, 46.7892) centre (144.78, 57.9553) ccw projected
  line L9 (150.8305, 46.7892) -> (207.094, 77.2765) projected
  arc A13 (238.76, 124.4818) -> (207.094, 77.2765) centre (225.385, 99.2303) ccw projected
  line L10 (238.76, 124.4818) -> (238.76, 169.0803) projected
  circle A14 centre (-99.2438, 137.3303) radius 14.2875 projected
  constraints: 4 end point, 2 point on circle
extrude "Extrusion7" [suppressed]
sketch "Sketch8" plane through (12.7, -57.9553, 48.26) normal (1, 0, 0) x (0, 0, -1)
  arc A0 (-123.1359, 156.0289) -> (-125.9731, 144.465) centre (-97.79, 143.6803) ccw
  line L0 (-122.8964, 163.3325) -> (-122.523, 159.4124)
  line L1 (-142.24, 169.0803) -> (-129.2178, 169.0803)
  spline S0 degree 2 poles (-221.2962, 144.7093) (-189.8396, 169.0803) (-142.24, 169.0803) knots 1 1 1 2 2 2
  arc A1 (-221.2962, 144.7093) -> (-187.7795, 106.6698) centre (-205.74, 124.6303) ccw
  spline S1 degree 3 poles (-159.7966, 136.4204) (-160.5161, 136.0307) (-162.9434, 134.6743) (-166.1744, 132.6857) (-170.3078, 129.9138) (-173.1321, 127.8669) (-175.1101, 126.3517) (-175.4939, 126.0547) knots 0 0 0 0 0.132459 0.448869 0.607074 0.923484 1 1 1 1
  spline S2 degree 3 poles (-180.582, 128.1282) (-180.5251, 127.7187) (-180.3887, 127.3243) (-179.9724, 126.6098) (-179.6965, 126.2967) (-179.0402, 125.7938) (-178.666, 125.6088) (-177.8679, 125.3927) (-177.4515, 125.3637) (-176.7607, 125.4505) (-176.4861, 125.5231) (-175.9633, 125.7391) (-175.7175, 125.8816) (-175.4939, 126.0547) knots 0 0 0 0 0.12403 0.12403 0.248059 0.248059 0.372089 0.372089 0.496118 0.496118 0.580963 0.580963 0.665808 0.665808 0.665808 0.665808
  arc A2 (-180.582, 128.1282) -> (-185.3963, 139.8386) centre (-205.74, 124.6303) ccw
  arc A3 (-182.4834, 144.893) -> (-185.3963, 139.8386) centre (-182.8533, 141.7397) ccw
  line L2 (-182.4834, 144.893) -> (-160.9387, 142.3656)
  spline S3 degree 3 poles (-159.7966, 136.4204) (-159.4331, 136.6173) (-159.1114, 136.8833) (-158.5883, 137.5236) (-158.3918, 137.8918) (-158.1509, 138.6828) (-158.1089, 139.0981) (-158.1864, 139.9213) (-158.3051, 140.3214) (-158.6893, 141.0536) (-158.9511, 141.3786) (-159.5039, 141.8425) (-159.7675, 142.0051) (-160.3334, 142.2494) (-160.6326, 142.3297) (-160.9387, 142.3656) knots 0 0 0 0 0.12403 0.12403 0.248059 0.248059 0.372089 0.372089 0.496118 0.496118 0.620148 0.620148 0.712599 0.712599 0.80505 0.80505 0.80505 0.80505
  line L3 (-150.5941, 147.5473) -> (-181.7868, 151.2066)
  spline S4 degree 3 poles (-182.3079, 157.4074) (-182.7047, 157.2914) (-183.0751, 157.099) (-183.7212, 156.583) (-183.9908, 156.2643) (-184.3926, 155.5417) (-184.521, 155.1446) (-184.6185, 154.3235) (-184.5865, 153.9073) (-184.3649, 153.1107) (-184.1773, 152.7379) (-183.6699, 152.085) (-183.3548, 151.8113) (-182.8106, 151.4993) (-182.6148, 151.4119) (-182.2086, 151.2779) (-181.9992, 151.2315) (-181.7868, 151.2066) knots 0 0 0 0 0.12403 0.12403 0.248059 0.248059 0.372089 0.372089 0.496118 0.496118 0.620148 0.620148 0.744178 0.744178 0.808342 0.808342 0.872507 0.872507 0.872507 0.872507
  spline S5 degree 3 poles (-182.3079, 157.4074) (-181.8014, 157.5555) (-180.2373, 158.0014) (-176.5127, 158.9811) (-172.1175, 159.9481) (-165.3484, 161.1597) (-158.303, 162.0566) (-152.1732, 162.4641) (-149.655, 162.5727) knots 0 0 0 0 0.050647 0.155729 0.365894 0.470976 0.786223 1 1 1 1
  spline S6 degree 3 poles (-146.3536, 159.1439) (-146.3201, 159.5559) (-146.3675, 159.9706) (-146.6185, 160.7584) (-146.8198, 161.1241) (-147.3511, 161.7576) (-147.6761, 162.0195) (-148.2892, 162.3414) (-148.5523, 162.438) (-149.097, 162.5599) (-149.3762, 162.5847) (-149.655, 162.5727) knots 0 0 0 0 0.12403 0.12403 0.248059 0.248059 0.372089 0.372089 0.45581 0.45581 0.539531 0.539531 0.539531 0.539531
  line L4 (-146.3536, 159.1439) -> (-147.0595, 150.4439)
  arc A4 (-150.5941, 147.5473) -> (-147.0595, 150.4439) centre (-150.2241, 150.7007) ccw
  arc A5 (-122.8964, 163.3325) -> (-129.2178, 169.0803) centre (-129.2178, 162.7303) ccw
  spline S7 degree 3 poles (-125.9731, 144.465) (-125.9961, 143.6384) (-126.1803, 142.8243) (-126.8505, 141.3124) (-127.33, 140.6292) (-128.4917, 139.516) (-129.1514, 139.0838) (-130.5947, 138.4809) (-131.3658, 138.3154) (-132.1476, 138.2941) knots 0 0 0 0 0.248059 0.248059 0.496118 0.496118 0.730735 0.730735 0.965351 0.965351 0.965351 0.965351
  arc A6 (-123.1359, 156.0289) -> (-122.523, 159.4124) centre (-128.8444, 158.8102) ccw
  spline S8 degree 3 poles (-132.1476, 138.2941) (-151.3774, 137.7699) (-171.7443, 122.7049) (-187.7795, 106.6698) knots 0.172109 0.172109 0.172109 0.172109 1 1 1 1
  circle A7 centre (-205.74, 124.6303) radius 15.24
  circle A8 centre (-133.9387, 147.2642) radius 1.27
  circle A9 centre (-131.9736, 159.9642) radius 1.27
  point P0 (48.26, 57.9553)
extrude "Extrusion8" [suppressed]
sketch "Sketch9" plane through (12.7, -57.9553, 48.26) normal (1, 0, 0) x (0, 0, -1)
  circle A0 centre (-133.9387, 147.2642) radius 3.175 projected
  circle A1 centre (-133.9387, 147.2642) radius 9.525
  circle A2 centre (-131.9736, 159.9642) radius 3.175 projected
  circle A3 centre (-131.9736, 159.9642) radius 9.525
  line L0 (238.76, 169.0803) -> (-142.24, 169.0803) projected
  line L1 (-142.24, 169.0803) -> (-143.4637, 147.2642)
  arc A4 (-83.6334, 81.0168) -> (-104.8264, 131.2456) centre (-126.8185, 92.3811) ccw projected
  spline S0 degree 4 poles (-133.9387, 137.7392) (-126.1967, 137.7392) (-117.8662, 144.9704) (-111.7841, 135.1827) (-104.8264, 131.2456) knots 0 0 0 0 0 1 1 1 1 1
  line L2 (238.76, 169.0803) -> (-142.24, 169.0803) projected
  circle A5 centre (144.78, 57.9553) radius 3.175 projected
  circle A6 centre (-48.26, 57.9553) radius 3.175 projected
  circle A7 centre (48.26, 57.9553) radius 3.175 projected
  circle A8 centre (-74.422, 103.9928) radius 3.175 projected
  circle A9 centre (-74.422, 78.5928) radius 3.175 projected
  circle A10 centre (81.2991, 80.8647) radius 2.0193 projected
  line L3 (-142.24, 169.0803) -> (-142.24, 124.4818) projected
  arc A11 (-110.574, 77.2765) -> (-142.24, 124.4818) centre (-128.865, 99.2303) ccw projected
  line L4 (-110.574, 77.2765) -> (-54.3105, 46.7892) projected
  arc A12 (-54.3105, 46.7892) -> (-42.2095, 46.7892) centre (-48.26, 57.9553) ccw projected
  line L5 (-42.2095, 46.7892) -> (-7.5631, 65.5629) projected
  arc A13 (7.5631, 65.5629) -> (-7.5631, 65.5629) centre (0, 51.6053) ccw projected
  line L6 (7.5631, 65.5629) -> (42.2095, 46.7892) projected
  arc A14 (42.2095, 46.7892) -> (54.3105, 46.7892) centre (48.26, 57.9553) ccw projected
  line L7 (54.3105, 46.7892) -> (88.9569, 65.5629) projected
  arc A15 (104.0831, 65.5629) -> (88.9569, 65.5629) centre (96.52, 51.6053) ccw projected
  line L8 (104.0831, 65.5629) -> (138.7295, 46.7892) projected
  arc A16 (138.7295, 46.7892) -> (150.8305, 46.7892) centre (144.78, 57.9553) ccw projected
  line L9 (150.8305, 46.7892) -> (207.094, 77.2765) projected
  arc A17 (238.76, 124.4818) -> (207.094, 77.2765) centre (225.385, 99.2303) ccw projected
  line L10 (238.76, 124.4818) -> (238.76, 169.0803) projected
  circle A18 centre (-99.2438, 137.3303) radius 14.2875 projected
  point P0 (-118.8733, 139.4546)
  point P1 (-126.0077, 152.539)
  point P2 (-134.7346, 169.0803)
  dimension "d72" = 19.05
  dimension "d73" = 19.05
  constraints: 2 centre point, 2 coincident, 2 end point, 2 point on circle, 5 other
  measures "d72" diameter of A1
  measures "d73" diameter of A3
extrude "Extrusion9" [suppressed]
extrude "Extrusion10" [suppressed]
extrude "Extrusion11" [suppressed]